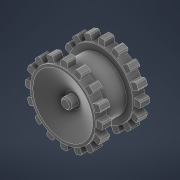
# Autodesk Inventor part: McCrea_front_wheel_walle
Saved by Autodesk Inventor 2022 (Build 260153000, 153)
## iProperties
Created: 2022-02-07
Part Number: McCrea_front_wheel_walle
Material: Generic
Document SubType Name: Modeling
Designer: student
Density: 1 g/cm^3
Appearance: Default
Author: student
Autodesk Inventor part; units mm, degrees
ref_plane "YZ Plane" through (0, 0, 0) normal (1, 0, 0) x (0, 1, 0)
ref_plane "XZ Plane" through (0, 0, 0) normal (0, 1, 0) x (-1, 0, 0)
sketch "Sketch1" plane through (0, 0, 0) normal (0, 0, 1) x (1, 0, 0)
  circle A0 centre (0, 0) radius 100
  dimension "d3" = 200
  constraints: 1 centre point, 1 coincident
  measures "d3" diameter of A0
extrude "Extrusion1" add sketch "Sketch1" along normal blind 50
sketch "Sketch2" plane through (0, 0, 50) normal (0, 0, 1) x (1, 0, 0)
  circle A0 centre (0, 0) radius 100 projected
  circle A1 centre (0, 0) radius 125
  dimension "d2" = 250
  constraints: 1 centre point
  measures "d2" diameter of A1
extrude "Extrusion2" add sketch "Sketch2" along normal blind 5 contours A0 | A1
sketch "Sketch3" plane through (0, 0, 55) normal (0, 0, 1) x (1, 0, 0)
  circle A0 centre (0, 0) radius 100 projected
  circle A1 centre (0, 0) radius 125 projected
  circle A2 centre (0, 0) radius 115
  dimension "d6" = 10
  constraints: 1 centre point, 1 coincident
  measures "d6" radial gap between concentric circles of A1 A2
extrude "Extrusion3" add sketch "Sketch3" along normal blind 40 contours A1
mirror "Mirror1" about plane through (0, 0, 0) normal (0, 0, 1) of "Extrusion1", "Extrusion3", "Extrusion2"
sketch "Sketch4" plane through (0, 0, 55) normal (0, 0, 1) x (1, 0, 0)
  circle A0 centre (0, 0) radius 20
  dimension "d9" = 40
  constraints: 1 centre point, 1 coincident
  measures "d9" diameter of A0
extrude "Extrusion4" add sketch "Sketch4" along normal blind 30
chamfer "Chamfer1" distance 40 angle 65 1 edges at (-115, 0, 55) measured on face at (114.8905, -5.0162, 81.6667)
ref_plane "Work Plane1" through (0, 0, 72.5) normal (0, 0, -1) x (-1, 0, 0)
sketch "Sketch6" plane through (0, 0, 72.5) normal (0, 0, -1) x (-1, 0, 0)
  circle A0 centre (0, 0) radius 125 projected
  line L0 (-124.3734, 12.5) -> (-145.3734, 12.5)
  line L1 (-149.3734, 8.5) -> (-149.3734, -8.5)
  line L2 (-145.3734, -12.5) -> (-124.3734, -12.5)
  line L3 (-124.3734, -12.5) -> (-124.3734, 12.5)
  line L4 (179.8747, 0) -> (-204.2481, 0) projected
  line L5 (-149.3734, -8.5) -> (-145.3734, -12.5)
  line L6 (-145.3734, 12.5) -> (-149.3734, 8.5)
  point P0 (-149.3734, -12.5)
  point P1 (-149.3734, 12.5)
  dimension "d15" = 25
  dimension "d16" = 25
  dimension "d17" = 4
  dimension "d18" = 4
  dimension "d19" = 4
  dimension "d20" = 4
  constraints: 12 end point, 4 point on line, 3 parallel, 2 point on circle, 1 horizontal, 1 perpendicular
  measures "d15" distance of point (-149.373, 12.5) point (-149.373, -12.5)
  measures "d16" distance of point (-149.373, -12.5) L2.end
  measures "d17" distance of L1.end point (-149.373, -12.5)
  measures "d18" distance of L2.start point (-149.373, -12.5)
  measures "d19" distance of L0.end point (-149.373, 12.5)
  measures "d20" distance of L1.start point (-149.373, 12.5)
extrude "Extrusion5" add sketch "Sketch6" along normal mid plane 35 contours A0 L4 L1 L6 L0 | L2 L5 L1 L4 A0
pattern_circular "Circular Pattern1" count 16 over 360 about axis through (0, 0, -10) along (0, 0, 1) of "Extrusion5"
mirror "Mirror2" about plane through (0, 0, 0) normal (0, 0, 1) of "Extrusion4", "Extrusion3", "Extrusion5", "Circular Pattern1", "Chamfer1", "Extrusion2"
sketch "Sketch7" plane through (0, 0, -55) normal (0, 0, -1) x (-1, 0, 0)
  circle A0 centre (0, 0) radius 29.2197 projected
  circle A1 centre (0, 0) radius 20 projected
extrude "Extrusion6" add sketch "Sketch7" along normal blind 60
chamfer "Chamfer2" distance 5 angle 45 1 edges at (-20, 0, 85)
equation "\"d18\" = d17"
equation "\"d19\" = d17"
equation "\"d20\" = d19"
body "Solid1"
